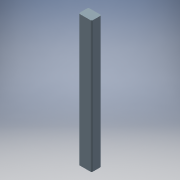
# Autodesk Inventor part: Product
Saved by Autodesk Inventor 2019 (Build 230136000, 136)
## iProperties
Created: 2017-01-18
Part Number: Product
Document SubType Name: Modeling
Designer: Administrator
Density: 1 g/cm^3
Mass: 59.3133 g
Surface Area: 139.064 cm^2
Volume: 59.3133 cm^3
Material: Generic
Appearance: Light Steel Blue
Author: Administrator
Autodesk Inventor part; units mm, degrees
ref_plane "YZ Plane" through (0, 0, 0) normal (1, 0, 0) x (0, 1, 0)
ref_plane "XZ Plane" through (0, 0, 0) normal (0, 1, 0) x (-1, 0, 0)
ref_plane "XY Plane" through (0, 0, 0) normal (0, 0, 1) x (1, 0, 0)
sketch "Sketch1" plane through (0, 0, 0) normal (0, 0, 1) x (1, 0, 0)
  line L0 (-10, -7.5) -> (10, -7.5)
  line L1 (10, -7.5) -> (10, 7.5)
  line L2 (10, 7.5) -> (-10, 7.5)
  line L3 (-10, 7.5) -> (-10, -7.5)
  line L4 (0, 0) -> (0, 7.5) construction
  line L5 (0, 0) -> (10, 0) construction
  line L6 (0, 0) -> (-10, 0) construction
  line L7 (0, 0) -> (0, -7.5) construction
  dimension "d0" = 20
  dimension "d1" = 15
  constraints: 16 end point, 4 midpoint, 4 perpendicular, 3 parallel, 2 collinear, 1 horizontal, 1 other
  measures "d0" distance of L1.end L2.end
  measures "d1" distance of L2.end L0.start
extrude "Extrusion1" add sketch "Sketch1" along normal mid plane 200
fillet "Fillet1" radius 2 4 edges at (10, -7.5, 0) (10, 7.5, 0) (-10, 7.5, 0) (-10, -7.5, 0)
body "Solid1"
